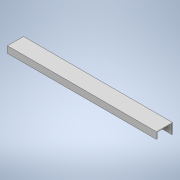
# Autodesk Inventor part: am-3920 AM14U
Saved by Autodesk Inventor 2020.3 (Build 243373000, 373)
## iProperties
Created: 2020-09-14
Part Number: am-3920 AM14U
Material: Generic
Document SubType Name: Modeling
Designer: super
Density: 1 g/cm^3
Appearance: Default
Author: super
Autodesk Inventor part; units mm, degrees
ref_plane "YZ Plane" through (0, 0, 0) normal (1, 0, 0) x (0, 1, 0)
ref_plane "XZ Plane" through (0, 0, 0) normal (0, 1, 0) x (-1, 0, 0)
ref_plane "XY Plane" through (0, 0, 0) normal (0, 0, 1) x (1, 0, 0)
sketch "Sketch1" plane through (0, 0, 0) normal (1, 0, 0) x (0, 1, 0)
  line L0 (0, 0) -> (0, 3.302)
  line L1 (0, 0) -> (53.975, 0)
  line L2 (53.975, 0) -> (53.975, 84.836)
  line L3 (53.975, 84.836) -> (19.05, 84.836)
  line L4 (19.05, 84.836) -> (19.05, 81.534)
  line L5 (19.05, 81.534) -> (50.673, 81.534)
  line L6 (50.673, 81.534) -> (50.673, 3.302)
  line L7 (50.673, 3.302) -> (0, 3.302)
  dimension "d0" = 3.302
  dimension "d1" = 53.975
  dimension "d2" = 84.836
  dimension "d3" = 34.925
  dimension "d4" = 3.302
  dimension "d5" = 31.623
  constraints: 16 end point, 6 perpendicular, 1 horizontal, 1 vertical
  measures "d0" distance of L0.start L0.end
  measures "d1" distance of L0.start L1.end
  measures "d2" distance of L1.end L2.end
  measures "d3" distance of L2.end L3.end
  measures "d4" distance of L3.end L4.end
  measures "d5" distance of L4.end L5.end
extrude "Extrusion1" add sketch "Sketch1" along normal blind 787.4
body "Solid1"
